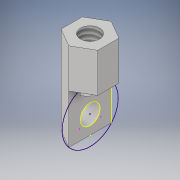
# Autodesk Inventor part: feet type 3 part 1 hexagon stock 10-32 hole
Saved by Autodesk Inventor 2018 (Build 220112000, 112)
## iProperties
Created: 2018-11-05
Part Number: feet type 3 part 1 hexagon stock 10-32 hole
Material: Generic
Document SubType Name: Modeling
Designer: Admin
Density: 1 g/cm^3
Appearance: Default
Author: Admin
Autodesk Inventor part; units mm, degrees
ref_plane "YZ Plane" through (0, 0, 0) normal (1, 0, 0) x (0, 1, 0)
ref_plane "XZ Plane" through (0, 0, 0) normal (0, 1, 0) x (-1, 0, 0)
ref_plane "XY Plane" through (0, 0, 0) normal (0, 0, 1) x (1, 0, 0)
sketch "Sketch1" plane through (0, 0, 0) normal (0, 1, 0) x (-1, 0, 0)
  line L0 (0, 0) -> (4.7625, 0)
  line L1 (4.7625, 0) -> (4.7625, -2.7496)
  line L2 (4.7625, 0) -> (7.5121, 0) construction
  line L3 (4.7625, 0) -> (4.7625, 2.7496)
  line L4 (2.3813, 4.1244) -> (0, 5.4993)
  line L5 (2.3813, 4.1244) -> (4.7625, 2.7496)
  line L6 (-2.3813, 4.1244) -> (-4.7625, 2.7496)
  line L7 (-2.3813, 4.1244) -> (0, 5.4993)
  line L8 (-4.7625, 0) -> (-4.7625, -2.7496)
  line L9 (-4.7625, 0) -> (-4.7625, 2.7496)
  line L10 (-2.3812, -4.1244) -> (0, -5.4993)
  line L11 (-2.3812, -4.1244) -> (-4.7625, -2.7496)
  line L12 (2.3813, -4.1244) -> (4.7625, -2.7496)
  line L13 (2.3813, -4.1244) -> (0, -5.4993)
  line L14 (4.7625, 2.7496) -> (4.7625, -2.7496)
  line L15 (4.7625, -2.7496) -> (0, -5.4993)
  line L16 (0, -5.4993) -> (-4.7625, -2.7496)
  line L17 (-4.7625, -2.7496) -> (-4.7625, 2.7496)
  line L18 (-4.7625, 2.7496) -> (0, 5.4993)
  line L19 (4.7625, 2.7496) -> (0, 5.4993)
  dimension "d0" = 4.7625
  dimension "d1" = 90
  dimension "d4" = 360
  constraints: 40 end point, 5 coincident, 2 horizontal, 2 point on line, 1 perpendicular, 1 symmetric about line, 1 vertical, 31 other
  measures "d0" distance of L0.start L0.end
  measures "d1" angle of L1 L2
extrude "Extrusion1" add sketch "Sketch1" along normal blind 22.86
sketch "Sketch2" plane through (0, 22.86, 0) normal (0, 1, 0) x (1, 0, 0)
  point P0 (0, 0)
  point P1 (0, 0)
  constraints: 1 coincident
hole "Hole1" at (0, 22.86, 0) direction (0, -1, 0) diameter 4.9784 depth 12.7 tip angle 118 thread size "1/4-20 UNC" class "2B" standard "ANSI Unified Screw Threads"
sketch "Sketch3" plane through (0, 0, 0) normal (0, -1, 0) x (1, 0, 0)
  line L0 (0, 0) -> (9.2843, 0)
  line L1 (9.2843, 0) -> (9.2843, -7.4131)
  line L2 (9.2843, -7.4131) -> (0, -7.4131)
  line L3 (0, -7.4131) -> (0, 0)
  line L4 (9.2843, 0) -> (9.2843, 7.4131)
  line L5 (9.2843, 7.4131) -> (0, 7.4131)
  line L6 (0, 7.4131) -> (0, 0)
  constraints: 14 end point, 2 parallel, 2 symmetric about line, 1 horizontal, 1 perpendicular
extrude "Extrusion2" cut sketch "Sketch3" against normal blind 12.7
sketch "Sketch5" plane through (0, 0, 5.4993) normal (1, 0, 0) x (0, 0, -1)
  line L0 (10.9985, 0) -> (10.9985, 12.7) projected
  line L1 (0, 0) -> (0, 12.7) projected
  line L2 (5.4993, 0) -> (5.4993, 4.7625)
  circle A0 centre (5.4993, 4.7625) radius 3.3782
  dimension "d17" = 4.7625
  dimension "d18" = 6.7564
  constraints: 2 end point, 1 centre point, 1 coincident, 1 vertical
  measures "d17" distance of L2.start L2.end
  measures "d18" diameter of A0
hole "Hole2" at (0, 4.7625, 0) direction (-1, 0, 0) diameter 5.1054 end through all clearance for "Flat Head Machine Screw (82)" size "#10" standard "Ansi Unified Screw Threads"
sketch "Sketch7" plane through (0, 0, 5.4993) normal (1, 0, 0) x (0, 0, -1)
  circle A0 centre (5.4993, 4.7625) radius 2.5527 projected
  line L0 (10.9985, 0) -> (10.9985, 12.7) projected
  circle A1 centre (5.4993, 4.7625) radius 7.2748
  point P0 (5.4993, 0)
  point P1 (2.7496, 2.7999)
  point P2 (8.2489, 2.7999)
  constraints: 1 coincident, 4 other
body "Solid1"
